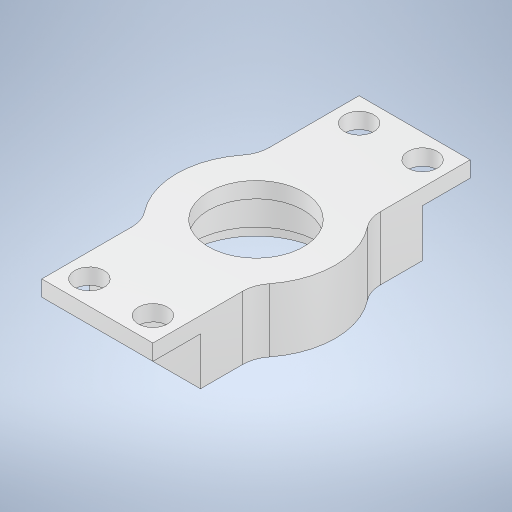
# Autodesk Inventor part: Shaft Brace
Saved by Autodesk Inventor 2023.2 (Build 272271000, 271)
## iProperties
Created: 2024-02-17
Part Number: Shaft Brace
Material: Aluminum 6061
Document SubType Name: Modeling
Designer: Nathan Cai
Density: 2.7 g/cm^3
Appearance: Aluminum - Flat
Author: Nathan Cai
Autodesk Inventor part; units mm, degrees
ref_plane "YZ Plane" through (0, 0, 0) normal (1, 0, 0) x (0, 1, 0)
ref_plane "XZ Plane" through (0, 0, 0) normal (0, 1, 0) x (-1, 0, 0)
ref_plane "XY Plane" through (0, 0, 0) normal (0, 0, 1) x (1, 0, 0)
sketch "Sketch1" plane through (0, 0, 0) normal (0, 1, 0) x (-1, 0, 0)
  circle A0 centre (0, 0) radius 6.35
  circle A1 centre (0, 0) radius 7.9375
  line L0 (5.5563, 15.875) -> (-5.5563, 15.875)
  line L1 (-5.5563, 15.875) -> (-5.5563, -15.875)
  line L2 (-5.5563, -15.875) -> (5.5563, -15.875)
  line L3 (5.5563, -15.875) -> (5.5563, 15.875)
  line L4 (5.5563, 15.875) -> (-5.5563, -15.875) construction
  line L5 (-5.5563, 15.875) -> (5.5563, -15.875) construction
  line L6 (-5.5563, 0) -> (5.5563, 0) construction
  line L7 (-5.5563, 15.875) -> (5.5563, 15.875)
  line L8 (5.5563, 15.875) -> (5.5563, 11.1125)
  line L9 (5.5563, 11.1125) -> (-5.5563, 11.1125)
  line L10 (-5.5563, 11.1125) -> (-5.5563, 15.875)
  line L11 (-5.5563, 13.4937) -> (5.5563, 13.4937) construction
  circle A2 centre (-3.175, 13.4937) radius 1.4732
  line L12 (0, 15.875) -> (0, 11.1125) construction
  circle A3 centre (3.175, 13.4937) radius 1.4732
  line L13 (5.5563, -15.875) -> (-5.5563, -15.875)
  line L14 (-5.5563, -15.875) -> (5.5563, -15.875)
  line L15 (5.5563, -15.875) -> (5.5563, -11.1125)
  line L16 (5.5563, -11.1125) -> (-5.5563, -11.1125)
  line L17 (-5.5563, -11.1125) -> (-5.5563, -15.875)
  line L18 (-5.5563, -13.4937) -> (5.5563, -13.4937) construction
  circle A4 centre (-3.175, -13.4937) radius 1.4732
  line L19 (0, -15.875) -> (0, -11.1125) construction
  circle A5 centre (3.175, -13.4937) radius 1.4732
  circle A6 centre (0, 0) radius 4.7625
  point P0 (-5.5563, 5.6685)
  point P1 (-5.5563, -5.6685)
  point P2 (5.5563, -5.6685)
  point P3 (5.5563, 5.6685)
  dimension "d0" = 12.7
  dimension "d1" = 15.875
  dimension "d2" = 11.1125
  dimension "d3" = 31.75
  dimension "d4" = 4.7625
  dimension "d5" = 2.9464
  dimension "d6" = 2.3813
  dimension "d7" = 9.525
  constraints: 40 end point, 11 symmetric about line, 8 midpoint, 7 centre point, 4 parallel, 3 coincident, 3 point on line, 2 horizontal, 2 perpendicular, 3 other
  measures "d0" diameter of A0
  measures "d1" diameter of A1
  measures "d2" distance of L2.end L1.end
  measures "d3" distance of L1.end L0.end
  measures "d4" distance of L7.end L8.end
  measures "d5" diameter of A2
  measures "d6" distance from line of L1 A2.centre
  measures "d7" diameter of A6
extrude "Extrusion1" add sketch "Sketch1" against normal blind 1.5875
extrude "Extrusion2" add sketch "Sketch1" against normal blind 6.35 contours A0 L3 A1 | A0 L1 A1 L3 | L3 A1 L1 A0 | A0 L1 A1 | A1 L1 L9 L3 | L3 L16 L1 A1
fillet "Fillet1" radius 3.175 4 edges at (-5.5563, -3.175, 5.6685) (-5.5563, -3.175, -5.6685) (5.5563, -3.175, 5.6685) (5.5563, -3.175, -5.6685)
sketch "Sketch2" plane through (0, -6.35, 0) normal (0, -1, 0) x (1, 0, 0)
  circle A0 centre (0, 0) radius 6.9453
  dimension "d13" = 13.8906
  constraints: 1 centre point, 1 coincident
  measures "d13" diameter of A0
extrude "Extrusion3" cut sketch "Sketch2" against normal blind 1.1906
body "Solid1"
